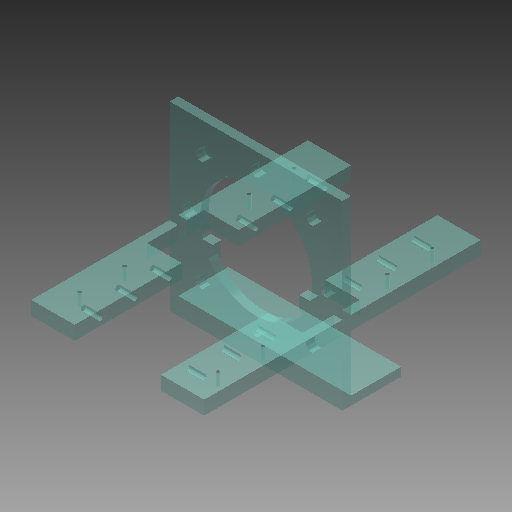
# Autodesk Inventor part: Base
Saved by Autodesk Inventor 2019 (Build 230136000, 136)
## iProperties
Created: 2017-01-18
Part Number: Base
Document SubType Name: Modeling
Designer: Administrator
Density: 1 g/cm^3
Mass: 101.625 g
Surface Area: 450.276 cm^2
Volume: 101.625 cm^3
Material: Generic
Appearance: Indoor Pool
Author: Administrator
Autodesk Inventor part; units mm, degrees
ref_plane "YZ Plane" through (0, 0, 0) normal (1, 0, 0) x (0, 1, 0)
ref_plane "XZ Plane" through (0, 0, 0) normal (0, 1, 0) x (-1, 0, 0)
sketch "Sketch1" plane through (0, 0, 0) normal (0, 0, 1) x (1, 0, 0)
  circle A0 centre (0, 0) radius 30 construction
  line L0 (0, 0) -> (0, 7.5) construction
  line L1 (0, 7.5) -> (10, 7.5) construction
  line L2 (10, 7.5) -> (10, 0) construction
  line L3 (10, 0) -> (0, 0) construction
  line L4 (0, 0) -> (-10, 0) construction
  line L5 (-10, 0) -> (-10, 7.5) construction
  line L6 (-10, 7.5) -> (0, 7.5) construction
  line L7 (-10, 0) -> (-10, -7.5) construction
  line L8 (-10, -7.5) -> (10, -7.5) construction
  line L9 (10, -7.5) -> (10, 0) construction
  circle A1 centre (-15.5891, 25.6316) radius 10 construction
  circle A2 centre (0, 0) radius 35 construction
  circle A3 centre (0, 0) radius 25 construction
  line L10 (0, 0) -> (-31.8198, 31.8198) construction
  circle A4 centre (0, 0) radius 45 construction
  line L11 (0, 0) -> (0, 45) construction
  circle A5 centre (0, 0) radius 40 construction
  circle A6 centre (-40, 0) radius 5 construction
  circle A7 centre (-31.8198, 31.8198) radius 10 construction
  line L12 (-31.8198, 31.8198) -> (-31.8198, -24.2384) construction
  line L13 (-31.8198, -24.2384) -> (-31.8198, -31.8198) construction
  circle A8 centre (-31.8198, -31.8198) radius 10 construction
  line L14 (-15, -20) -> (-15, -31.6228)
  line L15 (15, -20) -> (15, -31.6228)
  line L16 (-31.8198, 31.8198) -> (24.2384, 31.8198) construction
  line L17 (24.2384, 31.8198) -> (31.8198, 31.8198) construction
  line L18 (31.8198, 31.8198) -> (31.8198, -31.8198) construction
  line L19 (31.8198, -31.8198) -> (-31.8198, -31.8198) construction
  circle A9 centre (31.8198, 31.8198) radius 10 construction
  circle A10 centre (31.8198, -31.8198) radius 10 construction
  circle A11 centre (0, 40) radius 5 construction
  line L20 (0, 0) -> (40, 0) construction
  line L21 (0, 0) -> (0, -40) construction
  circle A12 centre (40, 0) radius 5 construction
  circle A13 centre (0, -40) radius 5 construction
  line L22 (50, 50) -> (50, -50)
  line L23 (50, -50) -> (-50, -50)
  line L24 (-50, -50) -> (-50, 50)
  line L25 (-50, 50) -> (50, 50)
  circle A14 centre (-31.8198, 31.8198) radius 3
  circle A15 centre (31.8198, 31.8198) radius 3
  circle A16 centre (31.8198, -31.8198) radius 3
  circle A17 centre (-31.8198, -31.8198) radius 3
  circle A18 centre (0, 0) radius 32.5
  point P0 (0, 50)
  dimension "d1" = 60
  dimension "d5" = 5
  dimension "d6" = 5
  dimension "d9" = 80
  dimension "d2" = 20
  dimension "d3" = 15
  dimension "d4" = 20
  dimension "d7" = 90
  dimension "d8" = 45
  dimension "d10" = 10
  dimension "d11" = 20
  dimension "d12" = 15
  dimension "d13" = 100
  dimension "d14" = 6
  dimension "d15" = 65
  constraints: 52 end point, 15 centre point, 14 coincident, 9 parallel, 7 perpendicular, 5 collinear, 5 point on circle, 3 equal radius, 2 point on line, 2 symmetric about line, 1 midpoint, 1 vertical, 32 other
  measures "d2" distance of L7.end L8.end
  measures "d3" distance between parallel lines of L8 L6
  measures "d4" diameter of A1
  measures "d7" diameter of A4
  measures "d8" angle of L11 L10
  measures "d10" diameter of A6
  measures "d11" diameter of A7
  measures "d12" distance between parallel lines of L14 L11
  measures "d13" distance of L22.start L22.end
  measures "d14" diameter of A14
  measures "d15" diameter of A18
extrude "Extrusion1" add sketch "Sketch1" against normal blind 5
sketch "Sketch2" plane through (50, -50, 0) normal (1, 0, 0) x (0, 0, -1)
  line L0 (0, 0) -> (5, 0) projected
  line L1 (5, 0) -> (34, 0)
  line L2 (5, 0) -> (0, 0)
  line L3 (0, 0) -> (0, -5)
  line L4 (0, -5) -> (34, -5)
  line L5 (34, -5) -> (34, 0)
  dimension "d18" = 29
  dimension "d27" = 5
  constraints: 10 end point, 3 perpendicular, 1 collinear, 1 horizontal
  measures "d18" distance of L0.end L1.end
  measures "d27" distance of L0.start L3.end
extrude "Extrusion2" add sketch "Sketch2" against normal up to surface (100 mm away)
ref_plane "Work Plane1" through (0, 0, 10.5) normal (0, 0, 1) x (1, 0, 0)
sketch "Sketch3" plane through (0, 0, 10.5) normal (0, 0, 1) x (1, 0, 0)
  line L0 (-8, -7.5) -> (8, -7.5)
  line L1 (10, -5.5) -> (10, 5.5)
  line L2 (8, 7.5) -> (-8, 7.5)
  line L3 (-10, 5.5) -> (-10, -5.5)
  arc A0 (-8, 7.5) -> (-10, 5.5) centre (-8, 5.5) ccw
  arc A1 (10, 5.5) -> (8, 7.5) centre (8, 5.5) ccw
  arc A2 (8, -7.5) -> (10, -5.5) centre (8, -5.5) ccw
  arc A3 (-10, -5.5) -> (-8, -7.5) centre (-8, -5.5) ccw
  point P0 (0, 0)
  point P1 (10, 7.5)
  point P2 (10, -7.5)
  point P3 (-10, 7.5)
  dimension "d22" = 20
  dimension "d23" = 15
  dimension "d24" = 7.5
  dimension "d25" = 10
  dimension "d26" = 2
  constraints: 8 end point, 8 point on circle, 8 tangent, 6 point on line, 4 centre point, 3 equal radius, 2 parallel, 1 horizontal, 1 perpendicular
  measures "d22" distance of point (10, 7.5) point (-10, 7.5)
  measures "d23" distance of point (10, -7.5) point (10, 7.5)
  measures "d24" distance from line of L2 point (0, 0)
  measures "d25" distance from line of L3 point (0, 0)
  measures "d26" radius of A0
sketch "Sketch4" plane through (0, 0, 0) normal (0, 0, 1) x (1, 0, 0)
  circle A0 centre (0, 0) radius 32.5 projected
  line L0 (50, -55) -> (-50, -55) projected
  line L1 (0, 0) -> (-32.5, 0) construction
  line L2 (0, 0) -> (0, -7.5) construction
  line L3 (0, -7.5) -> (-10, -7.5) construction
  line L4 (-10, -7.5) -> (-55, -7.5) construction
  line L5 (-50, -9.5) -> (-25, -9.5)
  line L6 (-25, -9.5) -> (-25, -17.5)
  line L7 (-25, -17.5) -> (-50, -17.5)
  line L8 (-50, -17.5) -> (-50, -9.5)
  line L9 (-25, -13.5) -> (-50, -13.5) construction
  line L10 (-50, 50) -> (-50, -55) projected
  dimension "d28" = 7.5
  dimension "d29" = 10
  dimension "d30" = 6
  dimension "d31" = 8
  dimension "d32" = 25
  dimension "d44" = 0
  constraints: 18 end point, 3 parallel, 3 perpendicular, 2 midpoint, 1 collinear, 1 horizontal, 1 horizontal alignment, 1 other
  measures "d28" distance between parallel lines of L1 L3
  measures "d29" distance of L2.end L3.end
  measures "d30" distance between parallel lines of L3 L9
  measures "d31" distance of L7.end L5.start
  measures "d32" distance between parallel lines of L6 L2
  measures "d44" distance between parallel lines of L8 L10
extrude "Extrusion3" add sketch "Sketch4" along normal blind 80 contours L5 L6 L7 A0 | A0 L7 L8 L5 picked at (-26.286, -13.9829)
sketch "Sketch5" plane through (-25, -17.5, 0) normal (1, 0, 0) x (0, 0, -1)
  line L0 (-80, 8) -> (-80, 0) projected
  line L1 (0, 4) -> (-80, 4) construction
  circle A0 centre (-25, 4) radius 1.5
  circle A1 centre (-45, 4) radius 1.5
  circle A2 centre (-65, 4) radius 1.5
  circle A3 centre (-25, 4) radius 6 construction
  circle A4 centre (-45, 4) radius 6 construction
  circle A5 centre (-65, 4) radius 6 construction
  line L2 (0, 67.5) -> (0, -37.5) projected
  dimension "d36" = 3
  dimension "d38" = 12
  dimension "d39" = 20
  dimension "d40" = 20
  dimension "d43" = 25
  constraints: 6 centre point, 4 equal radius, 3 coincident, 3 point on line, 2 end point, 1 midpoint
  measures "d36" diameter of A0
  measures "d38" diameter of A3
  measures "d39" distance of A1.centre A0.centre
  measures "d40" distance of A2.centre A1.centre
  measures "d43" distance from line of A0.centre L2
extrude "Extrusion4" cut sketch "Sketch5" against normal blind 10
mirror "Mirror1" about plane through (0, 0, 0) normal (1, 0, 0) of "Extrusion3", "Extrusion4"
mirror "Mirror2" about plane through (0, 0, 0) normal (0, 0, 1) of "Extrusion3", "Extrusion4", "Mirror1"
sketch "Sketch6" plane through (-50, -9.5, -5) normal (0, 1, 0) x (1, 0, 0)
  line L0 (18.9195, 0) -> (0, 0) construction
  line L1 (100, 0) -> (81.0805, 0) construction
  line L2 (100, 0) -> (100, 75) projected
  line L3 (100, 75) -> (75, 75) projected
  line L4 (0, 0) -> (25, 0)
  line L5 (25, 0) -> (25, 10)
  line L6 (25, 10) -> (0, 10) construction
  line L7 (0, 10) -> (0, 0) construction
  line L8 (75, 0) -> (100, 0)
  line L9 (100, 0) -> (100, 10) construction
  line L10 (100, 10) -> (75, 10) construction
  line L11 (75, 10) -> (75, 0)
  line L12 (5, 10) -> (5, 0)
  line L13 (95, 10) -> (95, 0)
  line L14 (95, 0) -> (75, 0)
  line L15 (75, 0) -> (75, 10)
  line L16 (75, 10) -> (95, 10)
  line L17 (95, 10) -> (95, 0)
  line L18 (5, 0) -> (25, 0)
  line L19 (25, 0) -> (25, 10)
  line L20 (25, 10) -> (5, 10)
  line L21 (5, 10) -> (5, 0)
  line L22 (100, -85) -> (75, -85) projected
  line L23 (100, -5) -> (100, -85) projected
  line L24 (81.0805, -5) -> (100, -5) projected
  line L25 (81.0805, 0) -> (81.0805, -5) projected
  line L26 (75, 75) -> (75, -85) projected
  line L27 (25, -85) -> (25, 75) projected
  dimension "d45" = 10
  dimension "d46" = 10
  dimension "d49" = 5
  dimension "d50" = 5
  dimension "d56" = 0
  dimension "d57" = 0
  constraints: 36 end point, 8 parallel, 6 perpendicular, 5 point on line, 4 horizontal
  measures "d45" distance between parallel lines of L6 L4
  measures "d46" distance between parallel lines of L10 L1
  measures "d49" distance between parallel lines of L13 L2
  measures "d50" distance between parallel lines of L7 L12
  measures "d56" distance between parallel lines of L27 L5
  measures "d57" distance between parallel lines of L26 L11
extrude "Extrusion5" cut sketch "Sketch6" against normal blind 10 contours L8 L11 L16 L13 | L12 L20 L5 L4
sketch "Sketch7" plane through (-50, -9.5, 0) normal (0, 1, 0) x (1, 0, 0)
  line L0 (0, 0) -> (18.9195, 0) projected
  line L1 (5, 0) -> (95, 0)
  line L2 (95, 0) -> (95, -18)
  line L3 (95, -18) -> (5, -18)
  line L4 (5, -18) -> (5, 0)
  line L5 (75, 80) -> (75, -80) projected
  line L6 (100, 0) -> (100, -80) projected
  line L7 (5, 5) -> (5, 15) projected
  line L8 (95, 15) -> (95, 5) projected
  point P0 (25, -80)
  point P1 (15, 0)
  point P2 (85, 0)
  dimension "d55" = 18
  dimension "d58" = 0
  dimension "d59" = 0
  constraints: 8 end point, 2 parallel, 1 horizontal, 1 perpendicular, 1 point on line, 2 other
  measures "d55" distance between parallel lines of L1 L3
  measures "d58" distance between parallel lines of L7 L4
  measures "d59" distance between parallel lines of L2 L8
extrude "Extrusion6" cut sketch "Sketch7" against normal blind 10
sketch "Sketch8" plane through (0, 0, 0) normal (0, 0, 1) x (1, 0, 0)
  line L0 (-31.0805, -9.5) -> (-25, -9.5) projected
  arc A0 (31.0805, -9.5) -> (-31.0805, -9.5) centre (0, 0) ccw projected
  circle A1 centre (0, 0) radius 40 construction
  line L1 (0, 0) -> (0, 40) construction
  circle A2 centre (0, 40) radius 3
  dimension "d61" = 80
  dimension "d60" = 6
  constraints: 2 coincident, 2 end point, 1 centre point, 1 perpendicular, 1 vertical alignment, 2 other
  measures "d60" diameter of A2
extrude "Extrusion7" cut sketch "Sketch8" against normal blind 10
pattern_circular "Circular Pattern1" count 4 over 360 about axis through (0, 0, 0) along (0, 0, -1) of "Extrusion7"
sketch "Sketch9" plane through (-50, -9.5, 80) normal (0, 1, 0) x (1, 0, 0)
  line L0 (0, 80) -> (0, 0) projected
  line L1 (12.5, 31) -> (0, 31) construction
  circle A0 centre (10, 44) radius 1
  circle A1 centre (10, 18) radius 1
  line L2 (18.9195, 80) -> (18.9195, 85) projected
  line L3 (10, 44) -> (10, 18) construction
  dimension "d67" = 2
  dimension "d68" = 13
  dimension "d69" = 13
  dimension "d72" = 10
  constraints: 4 end point, 2 centre point, 1 equal radius, 1 parallel, 1 perpendicular, 1 point on line, 1 other
  measures "d67" diameter of A0
  measures "d68" distance from line of L3.start L1
  measures "d69" distance from line of L3.end L1
  measures "d72" distance between parallel lines of L0 L3
extrude "Extrusion8" cut sketch "Sketch9" against normal blind 10
mirror "Mirror3" about plane through (0, 0, 0) normal (1, 0, 0) of "Extrusion8"
mirror "Mirror4" about plane through (0, 0, 0) normal (0, 0, 1) of "Extrusion8", "Mirror3"
body "Solid1"
